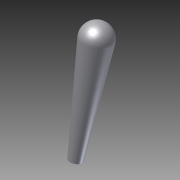
# Autodesk Inventor part: S_low_toggle
Saved by Autodesk Inventor 2011 SP1 (Build 150282100, 282)
## iProperties
Created: 2013-12-24
Part Number: S_low_toggle
Catalog Web Link: www.cadenas.de
Description: S Low Toggle-S Low Toggle
Vendor: NKKSWITCHES
Document SubType Name: Modeling
Designer: PARTuser1
Manufacturer: NKKSWITCHES
Density: 1 g/cm^3
Category: PARTsolutions
Company: NKKSWITCHES
Title: S_low_toggle
Author: Cadenas PARTsolutions
Comments: S Low Toggle
PSOL_IDENT_0: {$CADENAS_DATA\23d-libs\nkkswitches\toggle\s\parts\s_low_toggle.prj},172 {VTYP=3D},{NB=S_low_toggle}
PSOL_IDENT_1: ,{LINA=S_low_toggle},{NN=S Low Toggle},{DATE=05.04.2013 12:55:09},{GEOMDATE=05.04.2013 14:55:00},{VE
PSOL_IDENT_2: RSION=},{LINEID=10},{LINESUBID=-1},{WBVAR=}  {NB=S_low_toggle},{LINA=S_low_toggle},{KT=DUMMY},{PN=S_
PSOL_IDENT_3: low_toggle},{D=0.2400}
CNS_NN: S Low Toggle
CNS_NT: S Low Toggle
CNS_NB: S_low_toggle
CNS_NBSYN: $PN.
CNS_LINA: S_low_toggle
CNS_PN: S_low_toggle
CNS_D: 0.2400
SUPPLIER: NKKSWITCHES
ARTICLENO: S_low_toggle
BOMINFO: S_low_toggle
CREATOR: CADENAS GmbH
Autodesk Inventor part; units mm, degrees
sketch "Sketch_1" plane through (0, 0, 0) normal (1, 0, 0) x (0, 1, 0)
  line L0 (-1.1806, 0.8164) -> (22.5262, -4.4393)
  arc A0 (18.7155, -6.6543) -> (22.5262, -4.4393) centre (19.6001, -3.7906) ccw
  line L1 (18.7155, -6.6543) -> (-1.4555, -0.4235)
  line L2 (-1.4555, -0.4235) -> (-1.1806, 0.8164)
  line L3 (-1.1806, 0.8164) -> (22.5262, -4.4393)
  constraints: 8 end point, 2 point on circle, 1 centre point
revolve "Revolution1" add sketch "Sketch_1" angle 360 about axis through (0, -1.1806, 0.8164) along (0, 0.976296, -0.2164396)
ref_plane "toggle_XY" through (0, 2.5019, 0) normal (0, 1, 0) x (1, 0, 0)
ref_plane "toggle_YZ" through (0, 2.5019, 0) normal (1, 0, 0) x (0, 0, -1)
ref_plane "toggle_ZX" through (0, 2.5019, 0) normal (0, 0, -1) x (0, 1, 0)
ref_plane "toggle_cap_XY" through (0, 2.5019, 0) normal (0, -1, 0) x (1, 0, 0)
ref_plane "toggle_cap_YZ" through (0, 2.5019, 0) normal (1, 0, 0) x (0, 0, 1)
ref_plane "toggle_cap_ZX" through (0, 2.5019, 0) normal (0, 0, 1) x (0, -1, 0)
body "Solid1"
